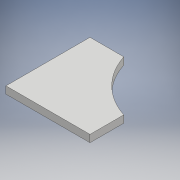
# Autodesk Inventor part: Naroznik_60x60
Saved by Autodesk Inventor 2018 (Build 220112000, 112)
## iProperties
Created: 2018-10-19
Part Number: Naroznik_60x60
Material: Ogólny
Document SubType Name: Modeling
Designer: EWA
Density: 1 g/cm^3
Appearance: Domyślna
Author: EWA
Autodesk Inventor part; units mm, degrees
ref_plane "YZ Plane" through (0, 0, 0) normal (1, 0, 0) x (0, 1, 0)
ref_plane "XZ Plane" through (0, 0, 0) normal (0, 1, 0) x (-1, 0, 0)
ref_plane "XY Plane" through (0, 0, 0) normal (0, 0, 1) x (1, 0, 0)
sketch "Szkic1" plane through (0, 0, 0) normal (0, 0, 1) x (1, 0, 0)
  line L0 (0, 0) -> (70, 0) construction
  line L1 (70, 0) -> (70, 70) construction
  line L2 (70, 70) -> (0, 70) construction
  line L3 (0, 70) -> (0, 0) construction
  line L4 (0, 0) -> (6, 0) construction
  line L5 (6, 0) -> (6, 70) construction
  line L6 (6, 70) -> (0, 70) construction
  line L7 (0, 70) -> (0, 0) construction
  line L8 (0, 0) -> (70, 0) construction
  line L9 (70, 0) -> (70, 6) construction
  line L10 (70, 6) -> (0, 6) construction
  line L11 (0, 6) -> (0, 0) construction
  line L12 (6, 6) -> (174, 6) construction
  line L13 (174, 6) -> (174, 174) construction
  line L14 (174, 174) -> (6, 174) construction
  line L15 (6, 174) -> (6, 6) construction
  line L16 (90, 174) -> (90, 6) construction
  circle A0 centre (90, 90) radius 65 construction
  line L17 (0, 0) -> (70, 0)
  line L18 (0, 0) -> (0, 70)
  line L19 (0, 70) -> (28.1534, 70)
  line L20 (70, 0) -> (70, 28.1534)
  arc A1 (28.1534, 70) -> (70, 28.1534) centre (90, 90) ccw
  dimension "d23" = 70
  dimension "d24" = 70
  dimension "d25" = 6
  dimension "d26" = 6
  dimension "d27" = 168
  dimension "d28" = 168
  dimension "d29" = 130
  constraints: 42 end point, 9 equal length, 6 point on line, 5 horizontal, 4 perpendicular, 4 point on circle, 3 midpoint, 2 centre point, 1 concentric
  measures "d23" distance of L2.end L1.end
  measures "d24" distance of L1.end L0.end
  measures "d25" distance of L6.end L5.end
  measures "d26" distance of L9.end L8.end
  measures "d27" distance of L14.end L13.end
  measures "d28" distance of L13.end L12.end
  measures "d29" diameter of A0
extrude "Wyciągnięcie proste1" add sketch "Szkic1" along normal blind 6
equation "\"d23\" = d24"
